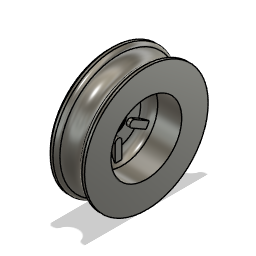
HyConiFlightXE2207PRO Source (Autodesk Fusion 360 design; units mm, degrees)
Autodesk Fusion 360 part; units mm, degrees
note: some values were not read from the file. Set by a fixed rule: which sketch regions a step uses.
other "Base Mesh Feature1"
other "Base Mesh Feature2"
sketch "Sketch1" plane through (0, 0, 0) normal (0, 1, 0) x (1, 0, 0)
  circle A0 centre (0, -25.5) radius 4.5
  line L0 (-8, -25.25) -> (-8, -14.45)
  line L1 (-8, -25.25) -> (-5.3644, -25.25)
  line L2 (-4.9679, -27.7601) -> (-4.4316, -24.7186)
  line L3 (-8, -14.45) -> (-6.7433, -14.45)
  line L4 (-6.7433, -14.45) -> (7, -14.45)
  line L5 (7, -14.45) -> (7, -25.25)
  line L6 (7, -25.25) -> (5.3644, -25.25)
  line L7 (4.4316, -24.7186) -> (5.123, -28.6395)
  line L8 (-8, -14.45) -> (-8, -3.05)
  line L9 (-6.2, -3.05) -> (-6.2, -4.8)
  line L10 (-6.2, -4.8) -> (-5.8, -4.8)
  line L11 (-5.8, -4.8) -> (-5.8, -10.45)
  circle A1 centre (-1.8, -10.45) radius 4
  line L12 (-8, -3.05) -> (-7.6, -2.65)
  line L13 (-7.6, -2.65) -> (-6.6, -2.65)
  line L14 (-6.6, -2.65) -> (-6.2, -3.05)
  line L15 (-5.3644, -25.25) -> (5.3644, -25.25)
  line L16 (-5.8, -10.45) -> (-5.8, -14.45) construction
  line L17 (-5.8, -14.45) -> (-2.8, -14.45) construction
  line L18 (-2.8, -14.45) -> (-2.8, -6.45) construction
  ellipse E0 centre (-2.8, -10.45) end of major axis (-2.8, -6.45) minor radius 3
  line L19 (-2.8, -14.45) -> (-2.8, -6.45)
  line L20 (0.2, -10.45) -> (-5.8, -10.45)
  dimension "d1" = 9
  dimension "d2" = 25.5
  dimension "d4" = 0.25
  dimension "d5" = 8
  dimension "d7" = 10
  dimension "d8" = 10
  dimension "d10" = 7
  dimension "d11" = 14.45
  dimension "d14" = 0.4
  dimension "d16" = 1
  dimension "d17" = 0.4
  dimension "d18" = 0.4
  dimension "d19" = 2.65
  dimension "d20" = 1.75
  dimension "d21" = 0.4
  dimension "d22" = 8
  dimension "d34" = 3
  dimension "d35" = 8
  constraint horizontal L1
  constraint coincident A0 L2.end
  constraint tangent A0 L2
  constraint vertical origin A0.centre
  constraint coincident L0.start L1.start
  constraint vertical L0
  constraint perpendicular L0 L3
  constraint perpendicular L0 L4
  constraint perpendicular L4 L5
  constraint perpendicular L5 L6
  constraint coincident A0 L7.start
  constraint horizontal L1.end L6.end
  constraint tangent A0 L7
  constraint perpendicular L3 L8
  constraint perpendicular L9 L10
  constraint perpendicular L10 L11
  constraint coincident L11.end A1
  constraint tangent L11 A1
  constraint tangent L4 A1
  constraint perpendicular L8 L13
  constraint vertical L9
  constraint horizontal L8.end L9.start
  constraint parallel L6 L15
  constraint coincident L4 L16.end
  constraint tangent A1 L16
  constraint perpendicular L16 L17
  constraint perpendicular L17 L18
  constraint coincident L17.end E0
  constraint coincident L18.end E0
  constraint coincident E0 L20.start
  constraint coincident L11.end E0
  measures "d1" diameter of A0
  measures "d2" distance of origin A0.centre
  measures "d4" distance of A0.centre L1
  measures "d5" distance of A0.centre L0
  measures "d7" angle of L0 L2
  measures "d8" angle of L5 L7
  measures "d10" horizontal distance of A0.centre L5.end
  measures "d11" distance of origin L4
  measures "d14" horizontal distance of L8.end L12.end
  measures "d16" distance of L12.end L13.end
  measures "d17" horizontal distance of L9.start L13.end
  measures "d18" vertical distance of L9.start L13.end
  measures "d19" distance of origin L13
  measures "d20" distance of L9.start L9.end
  measures "d21" distance of L9.end L10.end
  measures "d22" diameter of A1
  measures "d34" distance of L16.end L17.end
  measures "d35" distance of L17.end L18.end
revolve "Revolve1" add sketch "Sketch1" angle 360 about axis through (1.75, 0, 0) along (1, 0, 0) contours A0 L0 L1 L2 L3 L4 L5 L6 L7 L15 | L3 L4 L8 L9 L10 L11 L12 L13 L14 E0
sketch "Sketch2" plane through (-5.8, 0, 0) normal (1, 0, 0) x (0, 0, -1)
  circle A0 centre (0, 0) radius 4.8
  line L0 (1.35, 14.3868) -> (1.35, 6.9)
  line L1 (1.35, 6.9) -> (-1.35, 6.9)
  line L2 (-1.35, 6.9) -> (-1.35, 14.3868)
  circle A1 centre (0, 6.9) radius 1.35
  arc A2 (1.35, 14.3868) -> (-1.35, 14.3868) centre (0, 0) ccw
  circle A3 centre (0, 0) radius 14.45
  circle A4 centre (0, 0) radius 10.45
  dimension "d24" = 2.7
  dimension "d25" = 6.9
  constraint vertical L0
  constraint horizontal L1
  constraint vertical L2
  constraint midpoint L1 A1.centre
  constraint coincident L0.end A1
  constraint vertical A0.centre A1.centre
  constraint horizontal L2.end L0.start
  constraint coincident A0.centre A2.centre
  constraint coincident L2.end A3
  measures "d24" distance of L0.end L1.end
  measures "d25" distance of A0.centre A1.centre
extrude "Extrude1" add sketch "Sketch2" along normal blind 1.4 contours L0 L2 A2 A3 A4 | L0 L2 A1 A4 | L1 A1 | L1 A1 picked at (0.7648, 9.6531)
pattern_circular "C-Pattern1" count 6 over 360 about axis through (1.75, 0, 0) along (1, 0, 0) of "Extrude1"
fillet "Fillet1" radius 1.75 2 edges at (-4.5253, -9.1308, -23.5413) (4.5253, -9.1308, -23.5413)
chamfer "Chamfer1" distance 1 angle 45 1 edges at (-8, -9.1308, -23.5413)
equation "d8 = d7"
named bodies: "hy-con wheels iFlight XingE 2306 pro 10"
